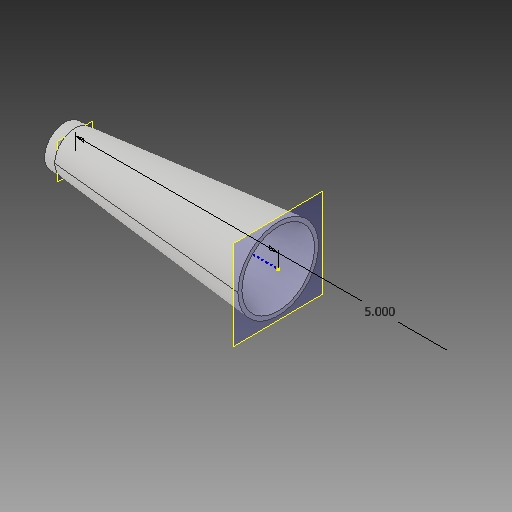
# Autodesk Inventor part: Gat to burner funnel
Saved by Autodesk Inventor 2019 (Build 230136000, 136)
## iProperties
Created: 2019-12-13
Part Number: Gat to burner funnel
Material: Generic
Document SubType Name: Modeling
Designer: Administrator
Density: 1 g/cm^3
Appearance: Default
Author: Administrator
Autodesk Inventor part; units mm, degrees
ref_plane "YZ Plane" through (0, 0, 0) normal (1, 0, 0) x (0, 1, 0)
ref_plane "XZ Plane" through (0, 0, 0) normal (0, 1, 0) x (-1, 0, 0)
ref_plane "XY Plane" through (0, 0, 0) normal (0, 0, 1) x (1, 0, 0)
ref_plane "Work Plane1" through (11.1704, -14409.1026, -14502.3728) normal (-0.9999676, 0.0015984, 0.0078835) x (0.0078813, -0.0013802, 0.999968)
sketch "Sketch1" plane through (11.1704, -14409.1026, -14502.3728) normal (-0.9999676, 0.0015984, 0.0078835) x (0.0078813, -0.0013802, 0.999968)
  circle A0 centre (0, 0) radius 25.4
  point P0 (14481.9337, 14428.8847)
  dimension "d0" = 50.8
  constraints: 1 centre point
  measures "d0" diameter of A0
sketch3d "3D Sketch2"
ref_plane "Work Plane2" through (-115.8296, -14409.1026, -14502.3728) normal (-1, 0, 0) x (0, -1, 0)
sketch "Sketch2" plane through (-115.8296, -14409.1026, -14502.3728) normal (-1, 0, 0) x (0, -1, 0)
  circle A0 centre (0, 0) radius 12.7
  point P0 (-14409.1026, 14502.3728)
  dimension "d2" = 25.4
  constraints: 1 centre point
  measures "d2" diameter of A0
loft "Loft1" add profiles "Sketch2", "Sketch1"
shell "Shell1" thickness 2.54 removed faces 2 at (-115.8296, -14408.7573, -14506.5337) at (11.1059, -14408.4119, -14510.6944)
sketch "Sketch3" plane through (-115.8296, -14409.1026, -14502.3728) normal (-1, 0, 0) x (0, 0, 1)
  line L0 (12.7, -0.0174) -> (25.3992, -0.0351) projected
  circle A0 centre (0, 0) radius 12.7
  circle A1 centre (0, 0) radius 10.16
  point P0 (14502.3728, 14409.1026)
  dimension "d8" = 20.32
  constraints: 1 centre point, 1 coincident, 3 other
  measures "d8" diameter of A1
extrude "Extrusion1" add sketch "Sketch3" along normal blind 6.35
body "Solid1"
